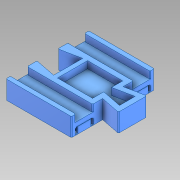
# Autodesk Inventor part: StraightRais-215
Saved by Autodesk Inventor 2021 (Build 250183000, 183)
## iProperties
Created: 2021-02-11
Part Number: StraightRais-215
Material: ABS プラスチック
Document SubType Name: Modeling
Designer: kumagai
Density: 1.06 g/cm^3
Appearance: 滑らか - 青
cp: 0.000 mm
ConnectorLength: 15.000 mm
RailWidth: 38.000 mm
JointFH: 9.500 mm
Author: kumagai
Autodesk Inventor part; units mm, degrees
ref_plane "YZ Plane" through (0, 0, 0) normal (1, 0, 0) x (0, 1, 0)
ref_plane "XZ Plane" through (0, 0, 0) normal (0, 1, 0) x (-1, 0, 0)
ref_plane "XY Plane" through (0, 0, 0) normal (0, 0, 1) x (1, 0, 0)
sketch "スケッチ1" plane through (0, 0, 0) normal (0, 1, 0) x (-1, 0, 0)
  line L0 (0, -26.6) -> (0, 26.6) projected
  line L1 (-31.8, 0) -> (22.8, 0) projected
  line L2 (15, -19) -> (-15, -19)
  line L3 (-15, 19) -> (15, 19)
  line L4 (15, -17) -> (-15, -17)
  line L5 (15, 17) -> (-15, 17)
  line L6 (15, -9.3) -> (-15, -9.3)
  line L7 (15, 9.3) -> (-15, 9.3)
  line L8 (-15, -4.7) -> (-24, -6.5)
  line L9 (-24, -6.5) -> (-24, 6.5)
  line L10 (-24, 6.5) -> (-15, 4.7)
  line L11 (-15, -19) -> (-15, -4.7)
  line L12 (-15, 4.7) -> (-15, 19)
  line L13 (15, -4.8) -> (5.5, -6.65)
  line L14 (5.5, -6.65) -> (5.5, 6.65)
  line L15 (5.5, 6.65) -> (15, 4.8)
  line L16 (15, 19) -> (15, 4.8)
  line L17 (15, -4.8) -> (15, -19)
  line L18 (3.5, -6.9) -> (-12.6, -6.9)
  line L19 (-12.6, 6.9) -> (3.5, 6.9)
  line L20 (3.5, 6.9) -> (3.5, -6.9)
  line L21 (-12.6, -1.7725) -> (-21.6, -3.5725)
  line L22 (-21.6, -3.5725) -> (-21.6, 3.5725)
  line L23 (-21.6, 3.5725) -> (-12.6, 1.7725)
  line L24 (-12.6, -6.9) -> (-12.6, -1.7725)
  line L25 (-12.6, 1.7725) -> (-12.6, 6.9)
  point P0 (0, 0)
  dimension "d0" = 38
  dimension "d2" = 9
  dimension "d3" = 13
  dimension "d4" = 30
  dimension "d5" = 9.4
  dimension "d6" = 2
  dimension "d7" = 18.6
  dimension "d8" = 9.5
  dimension "d9" = 9.6
  dimension "d10" = 13.3
  dimension "d11" = 2.4
  dimension "d12" = 2
  dimension "d13" = 2.4
  dimension "d14" = 2.4
  dimension "d15" = 2.4
  dimension "d24" = 2.4
  constraints: 48 end point, 12 parallel, 10 perpendicular, 8 point on line, 3 collinear, 2 horizontal, 2 vertical, 7 other
  measures "d0" distance between parallel lines of L3 L2
  measures "d2" distance between parallel lines of L9 L11
  measures "d3" distance of L9.end L8.end
  measures "d4" distance between parallel lines of L11 L17
  measures "d5" distance of L10.end L8.start
  measures "d6" distance between parallel lines of L2 L4
  measures "d7" distance between parallel lines of L7 L6
  measures "d8" distance between parallel lines of L14 L17
  measures "d9" distance of L15.end L13.start
  measures "d10" distance of L14.end L13.end
  measures "d11" distance between parallel lines of L18 L6
  measures "d12" distance between parallel lines of L14 L20
  measures "d13" distance between parallel lines of L11 L24
  measures "d14" distance between parallel lines of L9 L22
  measures "d15" distance between parallel lines of L10 L23
  measures "d24" distance between parallel lines of L21 L8
extrude "押し出し1" add sketch "スケッチ1" along normal blind 5.2 contours L4 L11 L6 L0 | L0 L6 L17 L4 | L18 L24 L21 L22 L1 L0 | L0 L1 L20 L18 | L1 L22 L23 L25 L19 L0 | L0 L19 L20 L1 | L7 L12 L5 L0 | L0 L5 L16 L7
extrude "押し出し2" add sketch "スケッチ1" along normal blind 8.4 contours L2 L11 L4 L0 | L0 L4 L17 L2 | L6 L11 L8 L9 L1 L22 L21 L24 L18 L0 | L0 L18 L20 L1 L14 L13 L17 L6 | L19 L25 L23 L22 L1 L9 L10 L12 L7 L0 | L0 L7 L16 L15 L14 L1 L20 L19 | L5 L12 L3 L0 | L0 L3 L16 L5
chamfer "面取り1" distance 0.4 angle 45 16 edges at (24, 4.2, 6.5) (24, 4.2, -6.5) (15, 4.2, -19) (15, 4.2, 19) (-15, 4.2, 19) (-15, 4.2, 4.8) (-15, 4.2, -4.8) (-15, 4.2, -19) (-15, 6.8, 9.3) (-15, 6.8, 17) (-15, 6.8, -9.3) (-15, 6.8, -17) (15, 6.8, -17) (15, 6.8, -9.3) (15, 6.8, 9.3) (15, 6.8, 17)
sketch "スケッチ2" plane through (0, 0, 0) normal (0, -1, 0) x (1, 0, 0)
  line L0 (0, 120.77) -> (0, -94.57) projected
  line L1 (-26.7776, 0) -> (29.6629, 0) projected
  line L2 (-4, 6.3) -> (4, 6.3)
  line L3 (4, 6.3) -> (4, 2.6)
  line L4 (4, 2.6) -> (-4, 2.6)
  line L5 (-4, 2.6) -> (-4, 6.3)
  line L6 (-4, -2.6) -> (4, -2.6)
  line L7 (4, -2.6) -> (4, -6.3)
  line L8 (4, -6.3) -> (-4, -6.3)
  line L9 (-4, -6.3) -> (-4, -2.6)
  line L10 (-15, 5.2) -> (-15, 18.6) projected
  line L11 (15, 18.6) -> (15, 4.7) projected
  line L12 (15, -4.7) -> (15, -18.6) projected
  line L13 (-15, -18.6) -> (-15, -5.2) projected
  line L14 (-18.7147, 13.1) -> (-16.9638, 13.1)
  line L15 (-15, 17.25) -> (-15, 8.95)
  line L16 (15, 17.25) -> (15, 8.95)
  arc A0 (0, 15.85) -> (-15, 17.25) centre (-15, -63.8071) ccw
  arc A1 (-15, 8.95) -> (0, 10.35) centre (-15, 90.0071) ccw
  arc A2 (15, 17.25) -> (0, 15.85) centre (15, -63.8071) ccw
  arc A3 (0, 10.35) -> (15, 8.95) centre (15, 90.0071) ccw
  line L17 (-0.005, 15.8509) -> (-0.005, 10.3491)
  line L18 (-0.005, 6.3) -> (-0.005, 2.6)
  line L19 (0.005, 15.8509) -> (0.005, 10.3491)
  line L20 (0.005, 6.3) -> (0.005, 2.6)
  point P0 (0, 0)
  point P1 (15, 8.95)
  dimension "d25" = 8
  dimension "d26" = 12.6
  dimension "d27" = 3.7
  dimension "d28" = 5.2
  dimension "d31" = 5.5
  dimension "d35" = 17.25
  dimension "d36" = 8.3
  dimension "d56" = 0.01
  constraints: 30 end point, 12 point on circle, 12 point on line, 5 symmetric about line, 4 centre point, 4 line through centre, 4 parallel, 4 vertical, 3 horizontal, 2 collinear, 2 perpendicular, 6 other
  measures "d25" distance between parallel lines of L3 L5
  measures "d26" distance between parallel lines of L8 L2
  measures "d27" distance between parallel lines of L2 L4
  measures "d28" distance between parallel lines of L6 L4
  measures "d31" distance of A1.end A0.start
  measures "d35" distance from line of L1 L16.start
  measures "d36" distance of L16.start L16.end
  measures "d56" distance between parallel lines of L19 L17
extrude "押し出し3" cut sketch "スケッチ2" against normal blind 3.2 contours L17 A1 L10 A0 | A2 L11 A3 L19 | L18 L4 L5 L2 | L2 L3 L4 L20
chamfer "面取り2" distance 0.6 angle 45 4 edges at (-7.4699, 3.2, 16.8995) (7.4699, 3.2, 16.8995) (-7.4699, 3.2, 9.3005) (7.4699, 3.2, 9.3005)
sketch "スケッチ3" plane through (0, 0, 0) normal (0, -1, 0) x (1, 0, 0)
  line L0 (-15, 9.55) -> (-15, 16.65) projected
  line L1 (-15, 17.35) -> (-14.7, 17.35)
  line L2 (-14.7, 8.85) -> (-15, 8.85)
  line L3 (-15, 8.85) -> (-15, 17.35)
  line L4 (-14.4, 15.5) -> (-0.5, 14.6)
  line L5 (-0.5, 11.6) -> (-14.4, 10.7)
  line L6 (-14.4, 17.05) -> (-14.4, 15.5)
  line L7 (-14.4, 14.999) -> (-14.4, 13.35)
  line L8 (-14.4, 12.85) -> (-14.4, 11.201)
  line L9 (-14.4, 10.7) -> (-14.4, 9.15)
  line L10 (-16.4042, 13.1) -> (-15.4023, 13.1)
  line L11 (0, 24.22) -> (0, -23.87) projected
  line L12 (-15, 16.15) -> (-14.4, 16.15)
  line L13 (-15, 10.05) -> (-14.4, 10.05)
  line L14 (-14.7, 17.35) -> (-14.4, 17.05)
  line L15 (-14.7, 8.85) -> (-14.4, 9.15)
  line L16 (-0.5, 14.099) -> (-0.8, 13.35)
  line L17 (-0.8, 12.85) -> (-0.5, 12.101)
  line L18 (-0.5, 12.101) -> (-0.5, 11.6)
  line L19 (-0.5, 14.099) -> (-0.5, 14.6)
  line L20 (-1.235, 14.1465) -> (-1.5541, 13.35)
  line L21 (-1.5541, 12.85) -> (-1.235, 12.0535)
  line L22 (-1.235, 14.1465) -> (-14.4, 14.999)
  line L23 (-14.4, 13.35) -> (-1.5541, 13.35)
  line L24 (-1.5541, 12.85) -> (-14.4, 12.85)
  line L25 (-14.4, 11.201) -> (-1.235, 12.0535)
  line L26 (-0.8, 13.35) -> (-0.8, 12.85)
  point P0 (0, 0)
  point P1 (-15, 17.25)
  point P2 (-15, 8.95)
  point P3 (-15, 16.15)
  point P4 (0, 15.35)
  point P5 (0, 10.85)
  point P6 (-15, 9.55)
  point P7 (-15, 16.65)
  dimension "d40" = 4.15
  dimension "d41" = 4.15
  dimension "d45" = 0.6
  dimension "d46" = 8.5
  dimension "d47" = 1.2
  dimension "d52" = 45
  dimension "d53" = 0.3
  dimension "d54" = 4.8
  dimension "d57" = 0.5
  dimension "d58" = 3
  dimension "d59" = 0.5
  dimension "d60" = 0.5
  dimension "d61" = 0.7
  dimension "d62" = 0.3
  constraints: 50 end point, 8 parallel, 8 point on line, 5 perpendicular, 4 horizontal, 3 collinear, 1 vertical, 9 other
  measures "d40" distance from line of L10 point (-15, 17.25)
  measures "d41" distance from line of L10 point (-15, 8.95)
  measures "d45" distance between parallel lines of L0 L7
  measures "d46" distance between parallel lines of L2 L1
  measures "d47" distance between parallel lines of L1 L12
  measures "d52" angle of L3 L14
  measures "d53" distance from line of L1.end L3
  measures "d54" distance of L5.end L4.start
  measures "d57" distance between parallel lines of L24 L23
  measures "d58" distance of L5.start L4.end
  measures "d59" distance between parallel lines of L22 L4
  measures "d60" distance from line of L4.end L11
  measures "d61" distance between parallel lines of L16 L20
  measures "d62" distance between parallel lines of L19 L26
extrude "押し出し4" add sketch "スケッチ3" against normal blind 3 contours L0 L12 L6 L4 L19 L16 L26 L17 L18 L5 L9 L13
extrude "押し出し5" add sketch "スケッチ3" against normal blind 0.4 contours L0 L13 L9 L15 L2 L3 | L0 L3 L1 L14 L6 L12
mirror "ミラー3" about plane through (0, 0, 0) normal (1, 0, 0) of "押し出し5", "押し出し4"
mirror "ミラー4" about plane through (0, 0, 0) normal (0, 0, 1) of "押し出し3", "面取り2", "押し出し4", "押し出し5", "ミラー3"
equation "\"d0\" = RailWidth"
equation "\"d2\" = JointMH"
equation "\"d3\" = JointMW1 - 2 * cp"
equation "\"d4\" = 2 * ConnectorLength"
equation "\"d5\" = JointMW2 - 2 * cp"
equation "\"d6\" = OuterWall"
equation "\"d7\" = InsideWidth"
equation "\"d8\" = JointFH"
equation "\"d9\" = JointFW2 + 2 * cp"
equation "\"d10\" = JointFW1 + 2 * cp"
equation "\"d11\" = InnerWall"
equation "\"d12\" = OuterWall"
equation "\"d13\" = InnerWall"
equation "\"d14\" = InnerWall"
equation "\"d15\" = InnerWall"
equation "\"d24\" = InnerWall"
equation "\"d17\" = RailHeight - RailDepth"
equation "\"d19\" = RailHeight"
equation "\"d33\" = RailDepth"
equation "\"d40\" = d41"
equation "\"rib\" = 0.5"
equation "\"gap\" = 0.2"
equation "\"RailWidth\" = 38"
equation "\"JointMH\" = 9"
equation "\"JointMW1\" = 13"
equation "\"cp\" = 0"
equation "\"ConnectorLength\" = 15"
equation "\"JointMW2\" = 9.4"
equation "\"OuterWall\" = 2"
equation "\"InsideWidth\" = 18.6"
equation "\"JointFH\" = 9.5"
equation "\"JointFW2\" = 9.6"
equation "\"JointFW1\" = 13.3"
equation "\"InnerWall\" = 2.4"
equation "\"RailHeight\" = 8.4"
equation "\"RailDepth\" = 3.2"
